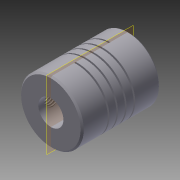
# Autodesk Inventor part: Acoplamiento elastico
Saved by Autodesk Inventor 2015 (Build 190159000, 159)
## iProperties
Created: 2013-02-24
Part Number: Acoplamiento elastico
Document SubType Name: Modeling
Designer: Lukas
Density: 1 g/cm^3
Mass: 6.05369 g
Surface Area: 47.5919 cm^2
Volume: 6.05369 cm^3
Material: Generic
Appearance: Aluminio mate
Author: Lukas
Autodesk Inventor part; units mm, degrees
ref_plane "XZ Plane" through (0, 0, 0) normal (0, 1, 0) x (-1, 0, 0)
ref_plane "XY Plane" through (0, 0, 0) normal (0, 0, 1) x (1, 0, 0)
sketch "Boceto1" plane through (0, 0, 0) normal (0, 0, 1) x (1, 0, 0)
  line L0 (-10, 12.5) -> (0, 12.5)
  line L1 (0, 12.5) -> (0, -12.5)
  line L2 (0, -12.5) -> (-10, -12.5)
  line L3 (-10, -12.5) -> (-10, 12.5)
  line L4 (-2.5, 12.5) -> (-2.5, 4.5)
  line L5 (-2.5, 4.5) -> (0, 4.5)
  line L6 (-2.5, -12.5) -> (-2.5, -4.5)
  line L7 (-2.5, -4.5) -> (0, -4.5)
  point P0 (0, 0)
  point P1 (0, 0)
  dimension "d0" = 20
  dimension "d1" = 25
  dimension "d2" = 8
  dimension "d3" = 8
  dimension "d4" = 5
  dimension "d5" = 5
  constraints: 16 end point, 4 perpendicular, 4 point on line, 3 parallel, 1 coincident, 1 horizontal, 1 midpoint
  measures "d0" diameter of L3 L1
  measures "d1" distance of L2.end L0.start
  measures "d2" distance of L6.start L6.end
  measures "d3" distance of L4.start L4.end
  measures "d4" diameter of L4 L1
  measures "d5" diameter of L6 L1
revolve "Revolución1" add sketch "Boceto1" angle 360 about axis through (0, 12.5, 0) along (0, -1, 0) contours L0 L4 L5 L1 L7 L6 L2 L3
sketch "Boceto2" plane through (0, 0, 0) normal (1, 0, 0) x (0, 1, 0)
  line L0 (12.5, -10) -> (12.5, 10) projected
  line L1 (-12.5, -10) -> (-12.5, 10) projected
  line L2 (12.5, -10) -> (12.5, 10) projected
  line L3 (-12.5, 0) -> (12.5, 0) construction
  line L4 (-5, 1.8114) -> (-4.5, 1.8114)
  line L5 (-4.5, 1.8114) -> (-4.5, 11.2321)
  line L6 (-4.5, 11.2321) -> (-5, 11.2321)
  line L7 (-5, 11.2321) -> (-5, 1.8114)
  dimension "d7" = 0.5
  dimension "d9" = 8
  constraints: 10 end point, 2 midpoint, 2 parallel, 1 horizontal, 1 perpendicular
  measures "d7" distance of L5.end L6.end
  measures "d9" distance between parallel lines of L1 L5
coil "Espira1" sketch "Boceto2" operation cut axis through (0, -12.5, 0) along (0, 1, 0) pitch 2.75 turns 4 hand right
sketch "Boceto3" plane through (0, 0, 0) normal (1, 0, 0) x (0, 1, 0)
  line L0 (-12.5, -2.5) -> (-12.5, 2.5) projected
  line L1 (12.5, -2.5) -> (12.5, 2.5) projected
  point P0 (-8.5, 0)
  point P1 (8.5, 0)
  point P2 (-12.5, 0)
  point P3 (12.5, 0)
  dimension "d18" = 4
  dimension "d19" = 4
  constraints: 2 horizontal alignment, 2 midpoint
  measures "d18" distance from line of L1 point (8.5, 0)
  measures "d19" distance from line of point (-8.5, 0) L0
hole "Agujero1" at (0, -8.5, 0) at (0, 8.5, 0) direction (-1, 0, 0) diameter 4.134 end through all thread size "M5x0.8" class "6H" standard "ISO Metric profile"
chamfer "Chaflán1" distance 0.5 angle 45 2 edges at (10, -12.5, 0) (10, 12.5, 0)
hole "Agujero2" at (0, -12.5, 0) direction (0, 1, 0) diameter 8 depth 19
equation "\"d19\" = d18"
equation "\"d3\" = d2"
equation "\"d5\" = d4"
body "Solid1"
